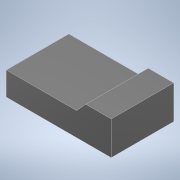
# Autodesk Inventor part: RC Reciever
Saved by Autodesk Inventor 2022 (Build 260153000, 153)
## iProperties
Created: 2022-08-09
Part Number: RC Reciever
Material: Generic
Document SubType Name: Modeling
Designer: Nick
Density: 1 g/cm^3
Appearance: Smooth - Black
Author: Nick
Autodesk Inventor part; units mm, degrees
ref_plane "YZ Plane" through (0, 0, 0) normal (1, 0, 0) x (0, 1, 0)
ref_plane "XZ Plane" through (0, 0, 0) normal (0, 1, 0) x (-1, 0, 0)
ref_plane "XY Plane" through (0, 0, 0) normal (0, 0, 1) x (1, 0, 0)
sketch "Sketch1" plane through (0, 0, 0) normal (0, 0, 1) x (1, 0, 0)
  line L0 (0, 0) -> (47, 0)
  line L1 (47, 0) -> (47, 15)
  line L2 (47, 15) -> (35.6, 15)
  line L3 (35.6, 15) -> (31.5, 10.5)
  line L4 (31.5, 10.5) -> (0, 10.5)
  line L5 (0, 10.5) -> (0, 0)
  dimension "d4" = 47
  dimension "d5" = 15
  dimension "d6" = 11.4
  dimension "d7" = 10.5
  dimension "d8" = 31.5
  constraints: 12 end point, 3 perpendicular, 1 horizontal, 1 parallel
  measures "d4" distance of L0.start L0.end
  measures "d5" distance of L0.end L1.end
  measures "d6" distance of L1.end L2.end
  measures "d7" distance of L4.end L0.start
  measures "d8" distance of L3.end L4.end
extrude "Extrusion1" add sketch "Sketch1" along normal blind 28
body "Solid1"
